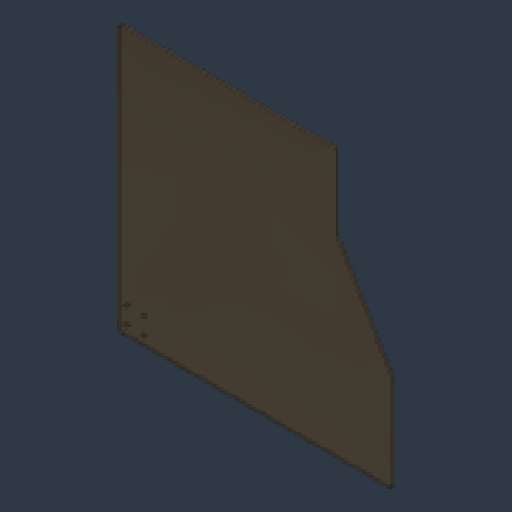
# Autodesk Inventor part: hopper_side_l
Saved by Autodesk Inventor 2024.3 (Build 283343000, 343)
## iProperties
Created: 2025-03-06
Part Number: hopper_side_l
Material: Polycarbonate, Smoke
Document SubType Name: Sheet Metal
Designer: marcu
Density: 1.2 g/cm^3
Sheet Metal Rule: Default
Appearance: Polycarbonate - Smoked
Author: marcu
Autodesk Inventor part; units mm, degrees
ref_plane "YZ Plane" through (0, 0, 0) normal (1, 0, 0) x (0, 1, 0)
ref_plane "XZ Plane" through (0, 0, 0) normal (0, 1, 0) x (-1, 0, 0)
ref_plane "XY Plane" through (0, 0, 0) normal (0, 0, 1) x (1, 0, 0)
sketch "Sketch1" plane through (0, 0, 0) normal (0, 0, 1) x (1, 0, 0)
  line L0 (203.2, -196.85) -> (-203.2, -196.85)
  line L1 (-203.2, -196.85) -> (-203.2, 196.85)
  line L2 (-203.2, 196.85) -> (203.2, 196.85)
  line L3 (203.2, 196.85) -> (203.2, -196.85)
  line L4 (203.2, -196.85) -> (-203.2, 196.85) construction
  line L5 (-203.2, -196.85) -> (203.2, 196.85) construction
  point P0 (0, 0)
  dimension "d0" = 406.4
  dimension "d1" = 393.7
  measures "d0" distance of L1.end L2.end
  measures "d1" distance of L0.end L1.end
extrude "Plate1" add sketch "Sketch1" along normal blind 3.048
sketch "Sketch2" plane through (0, 0, 3.048) normal (0, 0, 1) x (1, 0, 0)
  line L0 (203.2, 196.85) -> (203.2, -196.85) construction
  line L1 (-203.2, 196.85) -> (203.2, 196.85) construction
  line L2 (-203.2, -196.85) -> (-203.2, 196.85) construction
  line L3 (203.2, -196.85) -> (-203.2, -196.85) construction
  point P0 (0, 0)
  point P1 (-190.5, -184.15)
  point P2 (-165.1, -184.15)
  point P3 (-190.5, -158.75)
  point P4 (-165.1, -158.75)
  dimension "d3" = 12.7
  dimension "d4" = 12.7
  dimension "d7" = 25.4
  dimension "d10" = 25.4
  constraints: 1 horizontal, 1 vertical, 3 other
  measures "d3" distance from line of L3 point (-190.5, -184.15)
  measures "d4" distance from line of L2 point (-190.5, -184.15)
  measures "d7" distance of point (-190.5, -184.15) point (-165.1, -184.15)
  measures "d10" distance of point (-190.5, -184.15) point (-190.5, -158.75)
hole "Hole1" at (-190.5, -184.15, 3.048) at (-165.1, -184.15, 3.048) at (-190.5, -158.75, 3.048) at (-165.1, -158.75, 3.048) direction (0, 0, -1) diameter 5.1054 end through all clearance for "Flat Head Machine Screw (82)" size "#10" standard "Ansi Unified Screw Threads"
sketch "Sketch3" plane through (0, 0, 0) normal (0, 0, -1) x (-1, 0, 0)
  circle A0 centre (165.1, -158.75) radius 2.5527 construction
  circle A1 centre (190.5, -158.75) radius 2.5527 construction
  circle A2 centre (165.1, -184.15) radius 2.5527 construction
  circle A3 centre (190.5, -184.15) radius 2.5527 construction
  line L0 (-203.2, 196.85) -> (203.2, 196.85) projected
  line L1 (-203.2, -196.85) -> (-203.2, 196.85) projected
  line L2 (203.2, -196.85) -> (-203.2, -196.85) construction
  line L3 (203.2, 196.85) -> (203.2, -196.85) construction
  line L4 (-203.2, -57.15) -> (-56.553, 196.85)
  line L5 (-120.053, 86.8648) -> (-120.053, 196.85)
  point P0 (0, 0)
  dimension "d20" = 30
  dimension "d21" = 254
  dimension "d25" = 63.5
  constraints: 4 end point, 4 point on line, 1 perpendicular
  measures "d20" angle of L1 L4
  measures "d21" vertical distance of L4.start L4.end
  measures "d25" distance from line of L4.end L5
extrude "Cut1" cut sketch "Sketch3" against normal blind 3.048 contours L0 L5 L4 L1
fillet "Corner Round1" radius 6.35 6 edges at (203.2, -57.15, 1.524) (203.2, -196.85, 1.524) (-203.2, -196.85, 1.524) (-203.2, 196.85, 1.524) (120.053, 196.85, 1.524) (120.053, 86.8648, 1.524)
equation "\"d18\" = Thickness"
equation "\"d22\" = Thickness"
equation "\"d2\" = Thickness"
equation "\"BendRadius\" = Thickness"
equation "\"BendReliefWidth\" = Thickness"
equation "\"BendReliefDepth\" = 0.5 * Thickness"
equation "\"CornerReliefSize\" = 4 * Thickness"
equation "\"MinimumRemnant\" = 2 * Thickness"
equation "\"TransitionRadius\" = BendRadius"
equation "\"JacobiRadiusSize\" = BendRadius"
equation "\"GapSize\" = Thickness"
equation "\"Thickness\" = 3.048"
body "Solid1"
